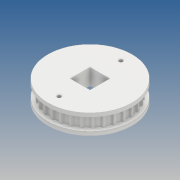
# Autodesk Inventor part: Poleas de transmision 30Dientes (ZR timing belts)
Saved by Autodesk Inventor 2020 (Build 240168000, 168)
## iProperties
Part Number: Poleas de transmision 30Dientes (ZR timing belts)
Material: Genérico
Document SubType Name: Modeling
Designer: FABLAB
Density: 1 g/cm^3
Appearance: Blanco
Description: Acrílico corte laser CNC
Author: FABLAB
Autodesk Inventor part; units mm, degrees
ref_plane "YZ Plane" through (0, 0, 0) normal (1, 0, 0) x (0, 1, 0)
ref_plane "XZ Plane" through (0, 0, 0) normal (0, 1, 0) x (-1, 0, 0)
ref_plane "XY Plane" through (0, 0, 0) normal (0, 0, 1) x (1, 0, 0)
sketch "Boceto1" plane through (0, 0, 0) normal (0, 0, 1) x (1, 0, 0)
  line L0 (8, -8) -> (-8, -8) projected
  line L1 (-8, -8) -> (-8, 8) projected
  line L2 (-8, 8) -> (8, 8) projected
  line L3 (8, 8) -> (8, -8) projected
  circle A0 centre (0, 0) radius 15 construction
  circle A1 centre (0, 0) radius 30
  circle A2 centre (0, 0) radius 25 construction
  circle A3 centre (0, 25) radius 1.5
  circle A4 centre (0, -25) radius 1.5
  circle A5 centre (0, 0) radius 31.2745 construction
  line L4 (-1.537, 29.9606) -> (1.537, 29.9606)
  line L5 (1.537, 29.9606) -> (0.9308, 31.2606)
  line L6 (0.9308, 31.2606) -> (-0.9308, 31.2606)
  line L7 (-0.9308, 31.2606) -> (-1.537, 29.9606)
  line L8 (0, 29.9606) -> (0, 0) construction
  line L9 (0, 0) -> (2.537, 29.8925) construction
  line L10 (0, 0) -> (-2.537, 29.8925) construction
  arc A6 (-2.537, 29.8925) -> (2.537, 29.8925) centre (0, 59.7851) ccw construction
  line L11 (1.537, 29.9606) -> (1.537, 32.0659) construction
  line L12 (-7.4099, 30.384) -> (-7.7325, 28.9863)
  line L13 (-5.589, 30.771) -> (-7.4099, 30.384)
  line L14 (-4.7258, 29.6254) -> (-5.589, 30.771)
  line L15 (-13.5651, 28.1794) -> (-13.5902, 26.7452)
  line L16 (-11.8645, 28.9366) -> (-13.5651, 28.1794)
  line L17 (-10.782, 27.9955) -> (-11.8645, 28.9366)
  line L18 (-19.1275, 24.7433) -> (-18.8538, 23.3352)
  line L19 (-17.6215, 25.8374) -> (-19.1275, 24.7433)
  line L20 (-16.367, 25.142) -> (-17.6215, 25.8374)
  line L21 (-23.854, 20.2257) -> (-23.2935, 18.9054)
  line L22 (-22.6084, 21.6091) -> (-23.854, 20.2257)
  line L23 (-21.2366, 21.1897) -> (-22.6084, 21.6091)
  line L24 (-27.5379, 14.8242) -> (-26.7151, 13.6492)
  line L25 (-26.6071, 16.4364) -> (-27.5379, 14.8242)
  line L26 (-25.1782, 16.3114) -> (-26.6071, 16.4364)
  line L27 (-30.0182, 8.7748) -> (-28.9692, 7.7966)
  line L28 (-29.443, 10.5453) -> (-30.0182, 8.7748)
  line L29 (-28.0193, 10.7201) -> (-29.443, 10.5453)
  line L30 (-31.1866, 2.342) -> (-29.9571, 1.6032)
  line L31 (-30.9921, 4.1933) -> (-31.1866, 2.342)
  line L32 (-29.6358, 4.6603) -> (-30.9921, 4.1933)
  line L33 (-30.9921, -4.1933) -> (-29.6358, -4.6603)
  line L34 (-31.1866, -2.342) -> (-30.9921, -4.1933)
  line L35 (-29.9571, -1.6032) -> (-31.1866, -2.342)
  line L36 (-29.443, -10.5453) -> (-28.0193, -10.7201)
  line L37 (-30.0182, -8.7748) -> (-29.443, -10.5453)
  line L38 (-28.9692, -7.7966) -> (-30.0182, -8.7748)
  line L39 (-26.6071, -16.4364) -> (-25.1782, -16.3114)
  line L40 (-27.5379, -14.8242) -> (-26.6071, -16.4364)
  line L41 (-26.7151, -13.6492) -> (-27.5379, -14.8242)
  line L42 (-22.6084, -21.6091) -> (-21.2366, -21.1897)
  line L43 (-23.854, -20.2257) -> (-22.6084, -21.6091)
  line L44 (-23.2935, -18.9054) -> (-23.854, -20.2257)
  line L45 (-17.6215, -25.8374) -> (-16.367, -25.142)
  line L46 (-19.1275, -24.7433) -> (-17.6215, -25.8374)
  line L47 (-18.8538, -23.3352) -> (-19.1275, -24.7433)
  line L48 (-11.8645, -28.9366) -> (-10.782, -27.9955)
  line L49 (-13.5651, -28.1794) -> (-11.8645, -28.9366)
  line L50 (-13.5902, -26.7452) -> (-13.5651, -28.1794)
  line L51 (-5.589, -30.771) -> (-4.7258, -29.6254)
  line L52 (-7.4099, -30.384) -> (-5.589, -30.771)
  line L53 (-7.7325, -28.9863) -> (-7.4099, -30.384)
  line L54 (0.9308, -31.2606) -> (1.537, -29.9606)
  line L55 (-0.9308, -31.2606) -> (0.9308, -31.2606)
  line L56 (-1.537, -29.9606) -> (-0.9308, -31.2606)
  line L57 (7.4099, -30.384) -> (7.7325, -28.9863)
  line L58 (5.589, -30.771) -> (7.4099, -30.384)
  line L59 (4.7258, -29.6254) -> (5.589, -30.771)
  line L60 (13.5651, -28.1794) -> (13.5902, -26.7452)
  line L61 (11.8645, -28.9366) -> (13.5651, -28.1794)
  line L62 (10.782, -27.9955) -> (11.8645, -28.9366)
  line L63 (19.1275, -24.7433) -> (18.8538, -23.3352)
  line L64 (17.6215, -25.8374) -> (19.1275, -24.7433)
  line L65 (16.367, -25.142) -> (17.6215, -25.8374)
  line L66 (23.854, -20.2257) -> (23.2935, -18.9054)
  line L67 (22.6084, -21.6091) -> (23.854, -20.2257)
  line L68 (21.2366, -21.1897) -> (22.6084, -21.6091)
  line L69 (27.5379, -14.8242) -> (26.7151, -13.6492)
  line L70 (26.6071, -16.4364) -> (27.5379, -14.8242)
  line L71 (25.1782, -16.3114) -> (26.6071, -16.4364)
  line L72 (30.0182, -8.7748) -> (28.9692, -7.7966)
  line L73 (29.443, -10.5453) -> (30.0182, -8.7748)
  line L74 (28.0193, -10.7201) -> (29.443, -10.5453)
  line L75 (31.1866, -2.342) -> (29.9571, -1.6032)
  line L76 (30.9921, -4.1933) -> (31.1866, -2.342)
  line L77 (29.6358, -4.6603) -> (30.9921, -4.1933)
  line L78 (30.9921, 4.1933) -> (29.6358, 4.6603)
  line L79 (31.1866, 2.342) -> (30.9921, 4.1933)
  line L80 (29.9571, 1.6032) -> (31.1866, 2.342)
  line L81 (29.443, 10.5453) -> (28.0193, 10.7201)
  line L82 (30.0182, 8.7748) -> (29.443, 10.5453)
  line L83 (28.9692, 7.7966) -> (30.0182, 8.7748)
  line L84 (26.6071, 16.4364) -> (25.1782, 16.3114)
  line L85 (27.5379, 14.8242) -> (26.6071, 16.4364)
  line L86 (26.7151, 13.6492) -> (27.5379, 14.8242)
  line L87 (22.6084, 21.6091) -> (21.2366, 21.1897)
  line L88 (23.854, 20.2257) -> (22.6084, 21.6091)
  line L89 (23.2935, 18.9054) -> (23.854, 20.2257)
  line L90 (17.6215, 25.8374) -> (16.367, 25.142)
  line L91 (19.1275, 24.7433) -> (17.6215, 25.8374)
  line L92 (18.8538, 23.3352) -> (19.1275, 24.7433)
  line L93 (11.8645, 28.9366) -> (10.782, 27.9955)
  line L94 (13.5651, 28.1794) -> (11.8645, 28.9366)
  line L95 (13.5902, 26.7452) -> (13.5651, 28.1794)
  line L96 (5.589, 30.771) -> (4.7258, 29.6254)
  line L97 (7.4099, 30.384) -> (5.589, 30.771)
  line L98 (7.7325, 28.9863) -> (7.4099, 30.384)
  point P0 (0, 31.2606)
  point P1 (-6.4994, 30.5775)
  point P2 (-12.7148, 28.558)
  point P3 (-18.3745, 25.2904)
  point P4 (-23.2312, 20.9174)
  point P5 (-27.0725, 15.6303)
  point P6 (-29.7306, 9.6601)
  point P7 (-31.0894, 3.2676)
  point P8 (-31.0894, -3.2676)
  point P9 (-29.7306, -9.6601)
  point P10 (-27.0725, -15.6303)
  point P11 (-23.2312, -20.9174)
  point P12 (-18.3745, -25.2904)
  point P13 (-12.7148, -28.558)
  point P14 (-6.4994, -30.5775)
  point P15 (0, -31.2606)
  point P16 (6.4994, -30.5775)
  point P17 (12.7148, -28.558)
  point P18 (18.3745, -25.2904)
  point P19 (23.2312, -20.9174)
  point P20 (27.0725, -15.6303)
  point P21 (29.7306, -9.6601)
  point P22 (31.0894, -3.2676)
  point P23 (31.0894, 3.2676)
  point P24 (29.7306, 9.6601)
  point P25 (27.0725, 15.6303)
  point P26 (23.2312, 20.9174)
  point P27 (18.3745, 25.2904)
  point P28 (12.7148, 28.558)
  point P29 (6.4994, 30.5775)
  dimension "d4" = 5
  dimension "d24" = 62.5489
  dimension "diametro" = 60
  dimension "d3" = 3
  dimension "d7" = 360
  dimension "d25" = 1.3
  dimension "d26" = 5.0739
  dimension "diente" = 5.08
  dimension "d28" = 25
  dimension "d29" = 50
  dimension "d30" = 3.0739
  dimension "d33" = 360
  constraints: 190 end point, 4 vertical alignment, 3 centre point, 3 coincident, 2 midpoint, 2 point on circle, 2 vertical, 1 equal length, 1 horizontal, 1 parallel, 258 other
  measures "d3" diameter of A3
  measures "d25" vertical distance of L4.end L5.end
  measures "d26" distance of L9.end L10.end
  measures "d28" angle of L8 L5
  measures "d29" angle of L5 L7
  measures "d30" distance of L4.end L4.start
extrude "Extrusión1" add sketch "Boceto1" along normal blind 10
sketch "Boceto2" plane through (0, 0, 0) normal (0, 0, -1) x (-1, 0, 0)
  circle A0 centre (0, 0) radius 34
  circle A1 centre (0, 0) radius 16
  circle A2 centre (0, 25) radius 1.5 projected
  circle A3 centre (0, -25) radius 1.5 projected
  circle A4 centre (0, -25) radius 1.5 construction
  circle A5 centre (0, -25) radius 9 construction
  dimension "d9" = 32
  dimension "d21" = 68
  constraints: 4 coincident, 3 centre point, 2 tangent
  measures "d9" diameter of A1
  measures "d21" diameter of A0
extrude "Extrusión2" add sketch "Boceto2" along normal blind 3 separate body
sketch "Boceto3" plane through (0, 0, 10) normal (0, 0, 1) x (1, 0, 0)
  circle A0 centre (0, 0) radius 34 projected
  circle A1 centre (0, 25) radius 1.5 projected
  circle A2 centre (0, -25) radius 1.5 projected
  line L0 (8, 8) -> (-8, 8) projected
  line L1 (8, -8) -> (8, 8) projected
  line L2 (-8, -8) -> (8, -8) projected
  line L3 (-8, 8) -> (-8, -8) projected
extrude "Extrusión3" add sketch "Boceto3" along normal blind 3 separate body
equation "\"diametro\" = 2 * dientes"
equation "\"dientes\" = 30"
